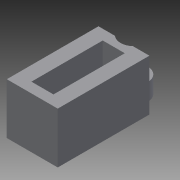
# Autodesk Inventor part: relay1
Saved by Autodesk Inventor 2013 (Build 170138000, 138)
## iProperties
Created: 2017-03-09
Part Number: relay1
Material: Generic
Document SubType Name: Modeling
Designer: Herman de Vries
Density: 1 g/cm^3
Author: Herman de Vries
Autodesk Inventor part; units mm, degrees
ref_plane "YZ Plane" through (0, 0, 0) normal (1, 0, 0) x (0, 1, 0)
ref_plane "XZ Plane" through (0, 0, 0) normal (0, 1, 0) x (-1, 0, 0)
ref_plane "XY Plane" through (0, 0, 0) normal (0, 0, 1) x (1, 0, 0)
sketch "Sketch1" plane through (0, 0, 0) normal (0, 0, 1) x (1, 0, 0)
  line L0 (0, 0) -> (15, 0)
  line L1 (15, 0) -> (15, 27)
  line L2 (15, 27) -> (0, 27)
  line L3 (0, 27) -> (0, 0)
  circle A0 centre (7.5, 30) radius 4
  circle A1 centre (7.5, 30) radius 1.5
  point P0 (7.5, 27)
  dimension "d2" = 15
  dimension "d3" = 27
  dimension "d7" = 8
  dimension "d8" = 3
  dimension "d9" = 3
  constraints: 8 end point, 2 centre point, 2 parallel, 1 coincident, 1 horizontal, 1 midpoint, 1 perpendicular, 1 vertical alignment
  measures "d2" distance of L0.start L0.end
  measures "d3" distance of L0.end L1.end
  measures "d7" diameter of A0
  measures "d8" distance from line of L2 A0.centre
  measures "d9" diameter of A1
extrude "Extrusion1" add sketch "Sketch1" along normal blind 15
sketch "Sketch2" plane through (0, 0, 15) normal (0, 0, 1) x (1, 0, 0)
  circle A0 centre (7.5, 30) radius 1.5
  line L0 (0, 27) -> (0, 0)
  line L1 (0, 0) -> (15, 0)
  line L2 (15, 0) -> (15, 27)
  circle A1 centre (7.5, 30) radius 4
  arc A2 (10.1458, 27) -> (4.8542, 27) centre (7.5, 30) ccw
  line L3 (4.25, 3) -> (10.75, 3)
  line L4 (10.75, 3) -> (10.75, 24)
  line L5 (10.75, 24) -> (4.25, 24)
  line L6 (4.25, 24) -> (4.25, 3)
  point P0 (11.4441, 29.3333)
  point P1 (3.5559, 29.3333)
  point P2 (10.75, 13.5)
  point P3 (15, 13.5)
  point P4 (7.5, 3)
  point P5 (7.5, 0)
  dimension "d14" = 6.5
  dimension "d16" = 21
  constraints: 14 end point, 4 midpoint, 3 centre point, 2 concentric, 2 parallel, 2 point on circle, 1 coincident, 1 horizontal, 1 horizontal alignment, 1 perpendicular, 1 vertical alignment
  measures "d14" distance of L3.start L3.end
  measures "d16" distance of L3.end L4.end
extrude "Extrusion2" cut sketch "Sketch2" against normal blind 10
fillet "Fillet2" radius 3 2 edges at (10.1458, 27, 2.5) (4.8542, 27, 2.5)
sketch "Sketch3" plane through (0, 0, 5) normal (0, 0, 1) x (1, 0, 0)
  line L0 (10.75, 3) -> (4.25, 3) construction
  line L1 (10.75, 24) -> (10.75, 3) construction
  line L2 (4.25, 24) -> (10.75, 24) construction
  line L3 (4.25, 3) -> (4.25, 24) construction
  line L4 (5.25, 23) -> (9.75, 23)
  line L5 (9.75, 23) -> (9.75, 4)
  line L6 (9.75, 4) -> (5.25, 4)
  line L7 (5.25, 4) -> (5.25, 23)
  point P0 (0, 0)
  dimension "d20" = 1
  constraints: 8 end point, 3 other
  measures "d20" distance between parallel lines of L2 L4
extrude "Extrusion3" cut sketch "Sketch3" against normal blind 10
body "Solid1"
